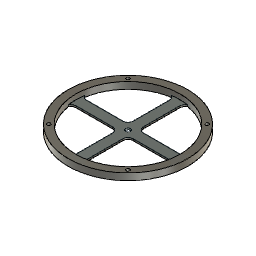
main_body_71mm_diameter v1 (Autodesk Fusion 360 design; units mm, degrees)
Autodesk Fusion 360 part; units mm, degrees
sketch "Sketch1" plane through (0, 0, 0) normal (0, 0, 1) x (1, 0, 0)
  circle A0 centre (0, 0) radius 36.5
  circle A1 centre (0, 0) radius 31.5
  line L0 (3, 0) -> (36.5, 0) construction
  circle A2 centre (-24.0416, 24.0416) radius 1
  circle A3 centre (24.0416, 24.0416) radius 1
  circle A4 centre (-24.0416, -24.0416) radius 1
  circle A5 centre (24.0416, -24.0416) radius 1
  line L1 (3, 6) -> (3, 27.8551)
  line L2 (-3, 27.8551) -> (-3, 6)
  line L3 (6, 3) -> (27.8715, 3)
  line L4 (27.8715, -3) -> (6, -3)
  line L5 (3, -6) -> (3, -27.8677)
  line L6 (3, -35) -> (-3, -35)
  line L7 (-3, -27.8677) -> (-3, -6)
  line L8 (-6, -3) -> (-27.8576, -3)
  line L9 (-27.8576, 3) -> (-6, 3)
  arc A6 (3, 6) -> (6, 3) centre (6, 6) ccw
  arc A7 (6, -3) -> (3, -6) centre (6, -6) ccw
  arc A8 (-3, -6) -> (-6, -3) centre (-6, -6) ccw
  arc A9 (-6, 3) -> (-3, 6) centre (-6, 6) ccw
  line L10 (-30.8224, 6.4582) -> (-30.7996, 6.6055)
  line L11 (-30.8224, -6.4582) -> (-30.7996, -6.6055)
  arc A10 (-30.8224, 6.4582) -> (-27.8576, 3) centre (-27.8576, 6) ccw
  arc A11 (-27.8576, -3) -> (-30.8224, -6.4582) centre (-27.8576, -6) ccw
  line L12 (-6.4497, -30.8338) -> (-6.43, -30.8367)
  line L13 (6.4497, -30.8338) -> (6.43, -30.8367)
  arc A12 (-6.4497, -30.8338) -> (-3, -27.8677) centre (-6, -27.8677) ccw
  arc A13 (3, -27.8677) -> (6.4497, -30.8338) centre (6, -27.8677) ccw
  line L14 (30.8381, 6.4465) -> (30.8507, 6.3627)
  line L15 (30.8381, -6.4465) -> (30.8507, -6.3627)
  arc A14 (30.8381, -6.4465) -> (27.8715, -3) centre (27.8715, -6) ccw
  arc A15 (27.8715, 3) -> (30.8381, 6.4465) centre (27.8715, 6) ccw
  line L16 (6.4603, 30.8195) -> (6.6494, 30.7902)
  line L17 (-6.4603, 30.8195) -> (-6.6494, 30.7902)
  arc A16 (-3, 27.8551) -> (-6.4603, 30.8195) centre (-6, 27.8551) ccw
  arc A17 (6.4603, 30.8195) -> (3, 27.8551) centre (6, 27.8551) ccw
  circle A18 centre (0, 0) radius 1.5
  dimension "d1" = 73
  dimension "d2" = 63
  dimension "d5" = 2
  dimension "d6" = 2
  dimension "d7" = 2
  dimension "d8" = 2
  dimension "d10" = 3
  dimension "d11" = 3
  dimension "d12" = 3
  dimension "d13" = 3
  dimension "d14" = 3
  dimension "d15" = 3
  dimension "d16" = 3
  dimension "d17" = 3
  dimension "d18" = 3
  dimension "d19" = 3
  dimension "d20" = 3
  dimension "d21" = 3
  dimension "d22" = 3
  constraint concentric A0 A1
  constraint horizontal L0
  constraint vertical L1
  constraint vertical L2
  constraint horizontal L3
  constraint horizontal L4
  constraint vertical L5
  constraint horizontal L6
  constraint vertical L7
  constraint horizontal L8
  constraint horizontal L9
  constraint coincident L0.start L1
  constraint tangent L1 A6
  constraint tangent L3 A6
  constraint tangent L4 A7
  constraint tangent L5 A7
  constraint tangent L8 A8
  constraint tangent L7 A8
  constraint tangent L9 A9
  constraint tangent L2 A9
  constraint coincident A1 L10.end
  constraint coincident A1 L11.end
  constraint tangent L10 A10
  constraint tangent L9 A10
  constraint tangent L11 A11
  constraint tangent L8 A11
  constraint coincident A1 L12.end
  constraint coincident A1 L13.end
  constraint coincident L6.end L7
  constraint tangent L12 A12
  constraint tangent L7 A12
  constraint coincident L6.start L5
  constraint tangent L5 A13
  constraint tangent L13 A13
  constraint coincident A1 L14.end
  constraint coincident A1 L15.end
  constraint tangent L15 A14
  constraint tangent L4 A14
  constraint tangent L3 A15
  constraint tangent L14 A15
  constraint coincident A1 L16.end
  constraint coincident A1 L17.end
  constraint tangent L17 A16
  constraint tangent L2 A16
  constraint tangent L16 A17
  constraint tangent L1 A17
  constraint concentric A0 A18
  measures "d1" diameter of A0
  measures "d2" diameter of A1
  measures "d5" diameter of A2
  measures "d6" diameter of A3
  measures "d7" diameter of A4
  measures "d8" diameter of A5
  measures "d10" radius of A6
  measures "d11" radius of A7
  measures "d12" radius of A8
  measures "d13" radius of A9
  measures "d14" radius of A10
  measures "d15" radius of A11
  measures "d16" radius of A12
  measures "d17" radius of A13
  measures "d18" radius of A14
  measures "d19" radius of A15
  measures "d20" radius of A16
  measures "d21" radius of A17
  measures "d22" diameter of A18
extrude "Extrude1" add sketch "Sketch1" along normal blind 1 contours A1 L1 L2 L3 L4 L5 L7 L8 L9 A6 A7 A8 A9 L10 L11 A10 A11 A12 A13 A14 A15 L16 L17 A16 A17
sketch "Sketch2" plane through (0, 0, 1) normal (0, 0, 1) x (-1, 0, 0)
  circle A0 centre (0, 0) radius 1.5
  arc A1 (-6.6494, -30.7902) -> (6.6494, -30.7902) centre (0, 0) ccw
  line L0 (6.6494, -30.7902) -> (6.4603, -30.8195)
  arc A2 (3, -27.8551) -> (6.4603, -30.8195) centre (6, -27.8551) ccw
  line L1 (3, -27.8551) -> (3, -6)
  arc A3 (6, -3) -> (3, -6) centre (6, -6) ccw
  line L2 (6, -3) -> (27.8576, -3)
  arc A4 (30.8224, -6.4582) -> (27.8576, -3) centre (27.8576, -6) ccw
  line L3 (30.8224, -6.4582) -> (30.7996, -6.6055)
  arc A5 (30.7996, -6.6055) -> (30.7996, 6.6055) centre (0, 0) ccw
  line L4 (30.7996, 6.6055) -> (30.8224, 6.4582)
  arc A6 (27.8576, 3) -> (30.8224, 6.4582) centre (27.8576, 6) ccw
  line L5 (27.8576, 3) -> (6, 3)
  arc A7 (3, 6) -> (6, 3) centre (6, 6) ccw
  line L6 (3, 6) -> (3, 27.8677)
  arc A8 (6.4311, 30.8365) -> (3, 27.8677) centre (6, 27.8677) ccw
  arc A9 (6.4311, 30.8365) -> (-6.4311, 30.8365) centre (0, 0) ccw
  arc A10 (-3, 27.8677) -> (-6.4311, 30.8365) centre (-6, 27.8677) ccw
  line L7 (-3, 27.8677) -> (-3, 6)
  arc A11 (-6, 3) -> (-3, 6) centre (-6, 6) ccw
  line L8 (-6, 3) -> (-27.8715, 3)
  arc A12 (-30.8477, 6.3774) -> (-27.8715, 3) centre (-27.8715, 6) ccw
  arc A13 (-30.8477, 6.3774) -> (-30.8477, -6.3774) centre (0, 0) ccw
  arc A14 (-27.8715, -3) -> (-30.8477, -6.3774) centre (-27.8715, -6) ccw
  line L9 (-27.8715, -3) -> (-6, -3)
  arc A15 (-3, -6) -> (-6, -3) centre (-6, -6) ccw
  line L10 (-3, -6) -> (-3, -27.8551)
  arc A16 (-6.4603, -30.8195) -> (-3, -27.8551) centre (-6, -27.8551) ccw
  line L11 (-6.4603, -30.8195) -> (-6.6494, -30.7902)
sketch "Sketch3" plane through (0, 0, 0) normal (0, 0, 1) x (1, 0, 0)
  circle A0 centre (0, 0) radius 31
  circle A1 centre (0, 0) radius 35.5
  line L0 (0, 0) -> (31, 0) construction
  circle A2 centre (-23.5113, 23.5113) radius 1
  circle A3 centre (23.5113, 23.5113) radius 1
  circle A4 centre (23.5113, -23.5113) radius 1
  circle A5 centre (-23.5113, -23.5113) radius 1
  arc A6 (23.5113, -23.5113) -> (24.2077, -22.7936) centre (0, 0) ccw
  dimension "d25" = 62
  dimension "d26" = 71
  dimension "d29" = 2
  dimension "d30" = 2
  dimension "d31" = 2
  dimension "d32" = 2
  constraint coincident A0.centre A1.centre
  constraint horizontal L0
  constraint coincident A4.centre A6.start
  constraint coincident A4 A6.end
  constraint coincident A0 L0.end
  measures "d25" diameter of A0
  measures "d26" diameter of A1
  measures "d29" diameter of A2
  measures "d30" diameter of A3
  measures "d31" diameter of A4
  measures "d32" diameter of A5
extrude "Extrude2" add sketch "Sketch3" along normal blind 4
